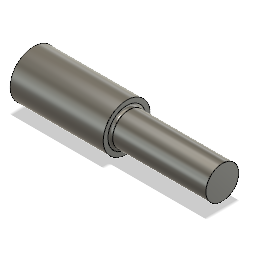
Table_17p1_Problem_17 (Autodesk Fusion 360 design; units mm, degrees)
Autodesk Fusion 360 part; units mm, degrees
sketch "Sketch1" plane through (0, 0, 0) normal (0, 0, 1) x (1, 0, 0)
  line L0 (0, 0) -> (0, 25)
  line L1 (0, 0) -> (200, 0)
  line L2 (200, 0) -> (200, 17.5)
  line L3 (200, 17.5) -> (101.25, 17.5)
  arc A0 (98.75, 20) -> (101.25, 17.5) centre (101.25, 20) ccw
  line L4 (98.75, 20) -> (98.75, 25)
  line L5 (98.75, 25) -> (0, 25)
  line L6 (0, 0) -> (0, -25) construction
  line L7 (98.75, -25) -> (0, -25) construction
  line L8 (200, 0) -> (200, -17.5) construction
  line L9 (200, -17.5) -> (101.25, -17.5) construction
  arc A1 (101.25, -17.5) -> (98.75, -20) centre (101.25, -20) ccw construction
  line L10 (98.75, -20) -> (98.75, -25) construction
  dimension "Shoulder_Height" = 7.5
  dimension "Fillet_Radius" = 2.5
  dimension "Bar_Length" = 200
  dimension "Bar_Diameter" = 50
  constraint coincident L0.start L1.start
  constraint vertical L0
  constraint perpendicular L0 L1
  constraint perpendicular L1 L2
  constraint perpendicular L2 L3
  constraint tangent L3 A0
  constraint perpendicular L3 L4
  constraint perpendicular L0 L5
  constraint equal L3 L5
  constraint tangent A0 L4
  constraint symmetric L0.start L1 L6.start
  constraint symmetric L0.end L1 L6.end
  constraint symmetric L2.start L1 L8.start
  constraint symmetric L1 L2.end L8.end
  constraint symmetric L1 L3.end L9.end
  constraint symmetric L1 A0.start A1.end
  constraint symmetric L1 A0 A1
  constraint symmetric L1 L4.end L7.start
  measures "Shoulder_Height" distance of L3 L5
  measures "Fillet_Radius" radius of A0
  measures "Bar_Length" distance of L0 L2
  measures "Bar_Diameter" distance of L5 L7
revolve "Revolve1" add sketch "Sketch1" angle 360 about axis through (0, 0, 0) along (1, 0, 0)
